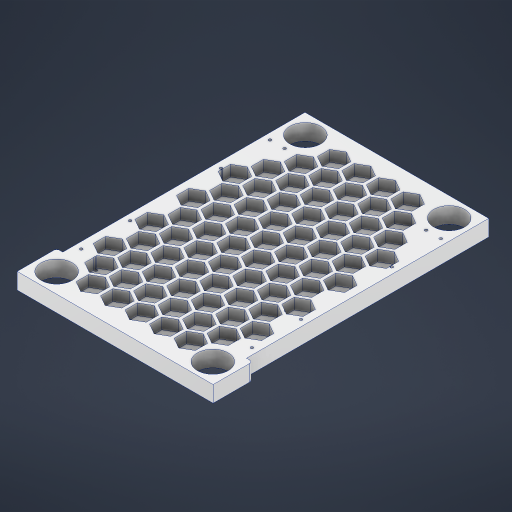
# Autodesk Inventor part: Weight Frame Top
Saved by Autodesk Inventor 2024 (Build 280153000, 153)
## iProperties
Created: 2022-10-18
Part Number: Weight Frame Top
Material: Aluminum 6061
Document SubType Name: Modeling
Designer: Hayden Swanson
Density: 2.7 g/cm^3
Appearance: Aluminum - Flat
Mass: 2392.19 g
Surface Area: 1313.96 cm^2
Volume: 885.998 cm^3
Author: Hayden Swanson
Autodesk Inventor part; units mm, degrees
ref_plane "YZ Plane" through (0, 0, 0) normal (1, 0, 0) x (0, 1, 0)
ref_plane "XZ Plane" through (0, 0, 0) normal (0, 1, 0) x (-1, 0, 0)
ref_plane "XY Plane" through (0, 0, 0) normal (0, 0, 1) x (1, 0, 0)
sketch "Sketch1" plane through (0, 0, 0) normal (0, 1, 0) x (-1, 0, 0)
  line L0 (0, 0) -> (190.5, 0)
  line L1 (190.5, 0) -> (190.5, -292.1)
  line L2 (190.5, -292.1) -> (0, -292.1)
  line L3 (0, -292.1) -> (0, 0)
  line L4 (0, -292.1) -> (-6.35, -292.1)
  line L5 (-6.35, -292.1) -> (-6.35, 0)
  line L6 (-6.35, 0) -> (0, 0)
  line L7 (190.5, -292.1) -> (196.85, -292.1)
  line L8 (196.85, -292.1) -> (196.85, 0)
  line L9 (196.85, 0) -> (190.5, 0)
  dimension "d0" = 190.5
  dimension "d1" = 292.1
  dimension "d259" = 6.35
  dimension "d260" = 6.35
  constraints: 20 end point, 4 perpendicular, 3 horizontal, 3 parallel
  measures "d0" distance of L1.end L2.end
  measures "d1" distance of L0.end L1.end
  measures "d259" distance of L2.end L4.end
  measures "d260" distance of L1.end L7.end
extrude "Extrusion1" add sketch "Sketch1" along normal blind 16.764
sketch "Sketch2" plane through (0, 16.764, 0) normal (0, 1, 0) x (1, 0, 0)
  line L0 (-176.2125, 0) -> (-176.2125, 20.32)
  line L1 (0, 0) -> (-14.2875, 0)
  line L2 (-14.2875, 0) -> (-14.2875, 20.32)
  line L3 (-190.5, 292.1) -> (-169.8625, 292.1)
  line L4 (-169.8625, 292.1) -> (-169.8625, 271.78)
  line L5 (-190.5, 271.78) -> (-190.5, 292.1)
  line L6 (0, 292.1) -> (-20.6375, 292.1)
  line L7 (-20.6375, 292.1) -> (-20.6375, 271.78)
  line L8 (0, 271.78) -> (0, 292.1)
  circle A0 centre (-176.2125, 20.32) radius 15.9766
  circle A1 centre (-14.2875, 20.32) radius 15.9766
  circle A2 centre (-20.6375, 271.78) radius 15.9766
  circle A3 centre (-169.8625, 271.78) radius 15.9766
  line L9 (6.35, 0) -> (6.35, 292.1) projected
  line L10 (6.35, 20.32) -> (-14.2875, 20.32)
  line L11 (-196.85, 292.1) -> (-196.85, 0) projected
  line L12 (-196.85, 20.32) -> (-176.2125, 20.32)
  dimension "d5" = 20.32
  dimension "d7" = 20.32
  dimension "d9" = 20.32
  dimension "d11" = 20.32
  dimension "d12" = 31.9532
  dimension "d14" = 31.9532
  dimension "d15" = 31.9532
  dimension "d264" = 31.9532
  dimension "d274" = 20.6375
  dimension "d276" = 20.6375
  constraints: 22 end point, 4 centre point, 4 coincident, 4 horizontal, 4 perpendicular, 2 parallel, 2 point on line
  measures "d5" distance of L0.end L0.start
  measures "d7" distance of L1.end L2.end
  measures "d9" distance of L3.end L4.end
  measures "d11" distance of L7.end L6.end
  measures "d12" diameter of A0
  measures "d14" diameter of A2
  measures "d15" diameter of A3
  measures "d264" diameter of A1
  measures "d274" distance of L10.start L10.end
  measures "d276" distance of L12.start L12.end
extrude "Extrusion2" cut sketch "Sketch2" against normal through all
sketch "Sketch7" plane through (0, 16.764, 0) normal (0, 1, 0) x (1, 0, 0)
  circle A0 centre (-14.2875, 20.32) radius 15.9766 projected
  line L0 (-14.2875, 53.2511) -> (-14.2875, 78.6511)
  line L1 (-14.2875, 78.6511) -> (-14.2875, 104.0511)
  line L2 (-14.2875, 53.2511) -> (-6.6675, 53.2511)
  line L3 (-14.2875, 104.0511) -> (-6.6675, 104.0511)
  line L4 (-14.2875, 104.0511) -> (-21.9075, 104.0511)
  line L5 (-14.2875, 53.2511) -> (-21.9075, 53.2511)
  line L6 (-14.2875, 198.2978) -> (-21.9075, 198.2978)
  line L7 (-14.2875, 249.0978) -> (-21.9075, 249.0978)
  line L8 (-14.2875, 198.2978) -> (-6.6675, 198.2978)
  line L9 (-14.2875, 249.0978) -> (-6.6675, 249.0978)
  circle A1 centre (-176.2125, 20.32) radius 15.9766 projected
  line L10 (-176.2125, 53.2511) -> (-176.2125, 78.6511)
  line L11 (-176.2125, 78.6511) -> (-176.2125, 104.0511)
  line L12 (-176.2125, 104.0511) -> (-176.2125, 198.2978)
  line L13 (-176.2125, 198.2978) -> (-176.2125, 223.6978)
  line L14 (-176.2125, 223.6978) -> (-176.2125, 249.0978)
  line L15 (-176.2125, 249.0978) -> (-168.5925, 249.0978)
  line L16 (-176.2125, 249.0978) -> (-183.8325, 249.0978)
  line L17 (-176.2125, 198.2978) -> (-183.8325, 198.2978)
  line L18 (-176.2125, 198.2978) -> (-168.5925, 198.2978)
  line L19 (-176.2125, 53.2511) -> (-183.8325, 53.2511)
  line L20 (-176.2125, 53.2511) -> (-168.5925, 53.2511)
  line L21 (-176.2125, 104.0511) -> (-183.8325, 104.0511)
  line L22 (-176.2125, 104.0511) -> (-168.5925, 104.0511)
  circle A2 centre (-183.8325, 53.2511) radius 1.75
  circle A3 centre (-183.8325, 104.0511) radius 1.75
  circle A4 centre (-168.5925, 53.2511) radius 1.75
  circle A5 centre (-168.5925, 104.0511) radius 1.75
  circle A6 centre (-183.8325, 198.2978) radius 1.75
  circle A7 centre (-168.5925, 198.2978) radius 1.75
  circle A8 centre (-183.8325, 249.0978) radius 1.75
  circle A9 centre (-168.5925, 249.0978) radius 1.75
  circle A10 centre (-21.9075, 53.2511) radius 1.75
  circle A11 centre (-6.6675, 53.2511) radius 1.75
  circle A12 centre (-21.9075, 104.0511) radius 1.75
  circle A13 centre (-6.6675, 104.0511) radius 1.75
  circle A14 centre (-21.9075, 198.2978) radius 1.75
  circle A15 centre (-21.9075, 249.0978) radius 1.75
  circle A16 centre (-6.6675, 198.2978) radius 1.75
  circle A17 centre (-6.6675, 249.0978) radius 1.75
  line L23 (-176.2125, 151.1745) -> (-14.2875, 151.1745)
  line L24 (-14.2875, 249.0978) -> (-14.2875, 53.2511)
  point P0 (0, 0)
  point P1 (6.35, 31.7989)
  point P2 (6.35, 8.8411)
  point P3 (-196.85, 8.8411)
  point P4 (-196.85, 31.7989)
  dimension "d167" = 25.4
  dimension "d168" = 25.4
  dimension "d169" = 94.2467
  dimension "d172" = 7.62
  dimension "d173" = 7.62
  dimension "d174" = 7.62
  dimension "d175" = 7.62
  dimension "d176" = 7.62
  dimension "d177" = 7.62
  dimension "d178" = 7.62
  dimension "d179" = 7.62
  dimension "d182" = 25.4
  dimension "d183" = 25.4
  dimension "d184" = 94.2467
  dimension "d185" = 25.4
  dimension "d186" = 25.4
  dimension "d187" = 7.62
  dimension "d188" = 7.62
  dimension "d189" = 7.62
  dimension "d190" = 7.62
  dimension "d191" = 7.62
  dimension "d192" = 7.62
  dimension "d193" = 7.62
  dimension "d194" = 7.62
  dimension "d195" = 3.5
  dimension "d196" = 3.5
  dimension "d197" = 3.5
  dimension "d198" = 3.5
  dimension "d199" = 3.5
  dimension "d200" = 3.5
  dimension "d201" = 3.5
  dimension "d202" = 3.5
  dimension "d203" = 3.5
  dimension "d204" = 3.5
  dimension "d205" = 3.5
  dimension "d206" = 3.5
  dimension "d207" = 3.5
  dimension "d208" = 3.5
  dimension "d209" = 3.5
  dimension "d210" = 3.5
  dimension "d258" = 161.925
  constraints: 50 end point, 16 centre point, 16 coincident, 14 horizontal, 4 point on line, 2 perpendicular, 1 midpoint, 2 other
  measures "d167" distance of L0.start L0.end
  measures "d168" distance of L0.end L1.end
  measures "d169" distance of L1.end L6.start
  measures "d172" distance of L0.start L2.end
  measures "d173" distance of L1.end L3.end
  measures "d174" distance of L1.end L4.end
  measures "d175" distance of L0.start L5.end
  measures "d176" distance of L6.start L6.end
  measures "d177" distance of L7.start L7.end
  measures "d178" distance of L6.start L8.end
  measures "d179" distance of L7.start L9.end
  measures "d182" distance of L10.start L10.end
  measures "d183" distance of L10.end L11.end
  measures "d184" distance of L11.end L12.end
  measures "d185" distance of L12.end L13.end
  measures "d186" distance of L13.end L14.end
  measures "d187" distance of L14.end L15.end
  measures "d188" distance of L14.end L16.end
  measures "d189" distance of L12.end L17.end
  measures "d190" distance of L12.end L18.end
  measures "d191" distance of L10.start L19.end
  measures "d192" distance of L10.start L20.end
  measures "d193" distance of L11.end L21.end
  measures "d194" distance of L11.end L22.end
  measures "d195" diameter of A2
  measures "d196" diameter of A3
  measures "d197" diameter of A4
  measures "d198" diameter of A5
  measures "d199" diameter of A6
  measures "d200" diameter of A7
  measures "d201" diameter of A8
  measures "d202" diameter of A9
  measures "d203" diameter of A10
  measures "d204" diameter of A11
  measures "d205" diameter of A12
  measures "d206" diameter of A13
  measures "d207" diameter of A14
  measures "d208" diameter of A15
  measures "d209" diameter of A16
  measures "d210" diameter of A17
  measures "d258" distance of L23.start L23.end
hole "Hole1" at (-183.8325, 16.764, -53.2511) at (-168.5925, 16.764, -53.2511) at (-183.8325, 16.764, -104.0511) at (-168.5925, 16.764, -104.0511) at (-183.8325, 16.764, -198.2978) at (-168.5925, 16.764, -198.2978) at (-183.8325, 16.764, -249.0978) at (-168.5925, 16.764, -249.0978) at (-6.6675, 16.764, -249.0978) at (-21.9075, 16.764, -249.0978) at (-6.6675, 16.764, -198.2978) at (-21.9075, 16.764, -198.2978) at (-6.6675, 16.764, -104.0511) at (-21.9075, 16.764, -104.0511) at (-6.6675, 16.764, -53.2511) at (-21.9075, 16.764, -53.2511) direction (0, -1, 0) diameter 2.85 end through all thread size "M3.5x0.6" class "6H" standard "ANSI Metric M Profile"
sketch "Sketch11" plane through (0, 16.764, 0) normal (0, 1, 0) x (1, 0, 0)
  circle A0 centre (-14.2875, 20.32) radius 15.9766 projected
  line L0 (-14.2875, 20.32) -> (-14.2875, 40.9575)
  line L1 (6.35, 292.1) -> (-196.85, 292.1) projected
  line L2 (6.35, 292.1) -> (0, 292.1)
  line L3 (0, 292.1) -> (0, 40.9575)
  line L4 (0, 40.9575) -> (6.35, 40.9575)
  line L5 (6.35, 40.9575) -> (6.35, 292.1)
  circle A1 centre (-176.2125, 20.32) radius 15.9766 projected
  line L6 (-176.2125, 20.32) -> (-176.2125, 40.9575)
  line L7 (-196.85, 292.1) -> (-196.85, 0) projected
  line L8 (-196.85, 292.1) -> (-190.5, 292.1)
  line L9 (-190.5, 292.1) -> (-190.5, 40.9575)
  line L10 (-190.5, 40.9575) -> (-196.85, 40.9575)
  line L11 (-196.85, 40.9575) -> (-196.85, 292.1)
  point P0 (0, 0)
  point P1 (-196.85, 40.9575)
  point P2 (6.35, 31.7989)
  point P3 (6.35, 8.8411)
  point P4 (-196.85, 8.8411)
  point P5 (-196.85, 31.7989)
  dimension "d266" = 20.6375
  dimension "d267" = 20.6375
  dimension "d272" = 6.35
  dimension "d273" = 6.35
  constraints: 20 end point, 4 parallel, 2 horizontal, 2 perpendicular, 2 vertical, 2 other
  measures "d266" distance of L0.start L0.end
  measures "d267" distance of L6.start L6.end
  measures "d272" distance of L3.end L4.end
  measures "d273" distance of L9.end L10.end
extrude "Extrusion10" cut sketch "Sketch11" against normal blind 16.764 contours L5 L4 L3 L1 | L9 L10 L7 L1
fillet "Fillet5" radius 3.175 2 edges at (-196.85, 8.382, -40.9575) (6.35, 8.382, -40.9575)
sketch "Sketch12" plane through (0, 16.764, 0) normal (0, 1, 0) x (1, 0, 0)
  line L0 (0, 292.1) -> (-190.5, 292.1) projected
  line L1 (0, 40.9575) -> (0, 292.1) projected
  arc A0 (-57.15, 292.1) -> (0, 234.95) centre (0, 292.1) ccw
  line L2 (-95.25, 316.441) -> (-95.25, -13.4796)
  line L3 (-232.3336, 146.05) -> (104.6921, 146.05)
  line L4 (-196.85, 0) -> (6.35, 0) projected
  arc A1 (-190.5, 234.95) -> (-133.35, 292.1) centre (-190.5, 292.1) ccw
  arc A2 (0, 57.15) -> (-57.15, 0) centre (0, 0) ccw
  arc A3 (-133.35, 0) -> (-190.5, 57.15) centre (-190.5, 0) ccw
  line L5 (-190.5, 234.95) -> (-190.5, 57.15)
  line L6 (-133.35, 0) -> (-57.15, 0)
  line L7 (0, 57.15) -> (0, 234.95)
  line L8 (-57.15, 292.1) -> (-133.35, 292.1)
  point P0 (0, 0)
  point P1 (-57.15, 0)
  dimension "d277" = 57.15
  dimension "d278" = 57.15
  dimension "d279" = 57.15
  dimension "d280" = 292.1
  dimension "d281" = 190.5
  dimension "d282" = 146.05
  dimension "d283" = 95.25
  constraints: 12 end point, 9 symmetric about line, 8 point on circle, 4 centre point, 3 collinear, 2 parallel, 2 point on line, 2 vertical, 1 horizontal, 3 other
  measures "d277" distance of L0.start L8.start
  measures "d278" distance of L0.start L7.end
  measures "d279" radius of A0
  measures "d280" distance between parallel lines of L0 L4
  measures "d281" distance of L0.end L0.start
  measures "d282" vertical distance of L0.end L3.start
  measures "d283" horizontal distance of L0.end L2.start
extrude "Extrusion11" [suppressed]
sketch "Sketch13" plane through (0, 16.764, 0) normal (0, 1, 0) x (1, 0, 0)
  line L0 (-160.4515, 34.036) -> (-160.4515, 21.336)
  line L1 (-160.4515, 21.336) -> (-171.45, 14.986)
  line L2 (-171.45, 14.986) -> (-182.4485, 21.336)
  line L3 (-182.4485, 21.336) -> (-182.4485, 34.036)
  line L4 (-182.4485, 34.036) -> (-171.45, 40.386)
  line L5 (-171.45, 40.386) -> (-160.4515, 34.036)
  line L6 (-190.5, 292.1) -> (-190.5, 40.9575) projected
  line L7 (-147.7515, 55.626) -> (-147.7515, 42.926)
  line L8 (-147.7515, 42.926) -> (-158.75, 36.576)
  line L9 (-158.75, 36.576) -> (-169.7485, 42.926)
  line L10 (-169.7485, 42.926) -> (-169.7485, 55.626)
  line L11 (-169.7485, 55.626) -> (-158.75, 61.976)
  line L12 (-158.75, 61.976) -> (-147.7515, 55.626)
  line L13 (-196.85, 0) -> (6.35, 0) projected
  line L14 (-147.7515, 86.106) -> (-158.75, 79.756)
  line L15 (-158.75, 79.756) -> (-169.7485, 86.106)
  line L16 (-147.7515, 98.806) -> (-147.7515, 86.106)
  line L17 (-169.7485, 86.106) -> (-169.7485, 98.806)
  line L18 (-169.7485, 98.806) -> (-158.75, 105.156)
  line L19 (-158.75, 105.156) -> (-147.7515, 98.806)
  line L20 (-182.4485, 77.216) -> (-171.45, 83.566)
  line L21 (-160.4515, 77.216) -> (-160.4515, 64.516)
  line L22 (-182.4485, 64.516) -> (-182.4485, 77.216)
  line L23 (-160.4515, 64.516) -> (-171.45, 58.166)
  line L24 (-171.45, 58.166) -> (-182.4485, 64.516)
  line L25 (-171.45, 83.566) -> (-160.4515, 77.216)
  line L26 (-147.7515, 129.286) -> (-158.75, 122.936)
  line L27 (-158.75, 122.936) -> (-169.7485, 129.286)
  line L28 (-147.7515, 141.986) -> (-147.7515, 129.286)
  line L29 (-169.7485, 129.286) -> (-169.7485, 141.986)
  line L30 (-169.7485, 141.986) -> (-158.75, 148.336)
  line L31 (-158.75, 148.336) -> (-147.7515, 141.986)
  line L32 (-182.4485, 120.396) -> (-171.45, 126.746)
  line L33 (-160.4515, 120.396) -> (-160.4515, 107.696)
  line L34 (-182.4485, 107.696) -> (-182.4485, 120.396)
  line L35 (-160.4515, 107.696) -> (-171.45, 101.346)
  line L36 (-171.45, 101.346) -> (-182.4485, 107.696)
  line L37 (-171.45, 126.746) -> (-160.4515, 120.396)
  line L38 (-147.7515, 172.466) -> (-158.75, 166.116)
  line L39 (-158.75, 166.116) -> (-169.7485, 172.466)
  line L40 (-147.7515, 185.166) -> (-147.7515, 172.466)
  line L41 (-169.7485, 172.466) -> (-169.7485, 185.166)
  line L42 (-169.7485, 185.166) -> (-158.75, 191.516)
  line L43 (-158.75, 191.516) -> (-147.7515, 185.166)
  line L44 (-182.4485, 163.576) -> (-171.45, 169.926)
  line L45 (-160.4515, 163.576) -> (-160.4515, 150.876)
  line L46 (-182.4485, 150.876) -> (-182.4485, 163.576)
  line L47 (-160.4515, 150.876) -> (-171.45, 144.526)
  line L48 (-171.45, 144.526) -> (-182.4485, 150.876)
  line L49 (-171.45, 169.926) -> (-160.4515, 163.576)
  line L50 (-147.7515, 215.646) -> (-158.75, 209.296)
  line L51 (-158.75, 209.296) -> (-169.7485, 215.646)
  line L52 (-147.7515, 228.346) -> (-147.7515, 215.646)
  line L53 (-169.7485, 215.646) -> (-169.7485, 228.346)
  line L54 (-169.7485, 228.346) -> (-158.75, 234.696)
  line L55 (-158.75, 234.696) -> (-147.7515, 228.346)
  line L56 (-182.4485, 206.756) -> (-171.45, 213.106)
  line L57 (-160.4515, 206.756) -> (-160.4515, 194.056)
  line L58 (-182.4485, 194.056) -> (-182.4485, 206.756)
  line L59 (-160.4515, 194.056) -> (-171.45, 187.706)
  line L60 (-171.45, 187.706) -> (-182.4485, 194.056)
  line L61 (-171.45, 213.106) -> (-160.4515, 206.756)
  line L62 (-122.3515, 42.926) -> (-133.35, 36.576)
  line L63 (-133.35, 36.576) -> (-144.3485, 42.926)
  line L64 (-122.3515, 55.626) -> (-122.3515, 42.926)
  line L65 (-144.3485, 42.926) -> (-144.3485, 55.626)
  line L66 (-144.3485, 55.626) -> (-133.35, 61.976)
  line L67 (-133.35, 61.976) -> (-122.3515, 55.626)
  line L68 (-157.0485, 34.036) -> (-146.05, 40.386)
  line L69 (-135.0515, 34.036) -> (-135.0515, 21.336)
  line L70 (-157.0485, 21.336) -> (-157.0485, 34.036)
  line L71 (-135.0515, 21.336) -> (-146.05, 14.986)
  line L72 (-146.05, 14.986) -> (-157.0485, 21.336)
  line L73 (-146.05, 40.386) -> (-135.0515, 34.036)
  line L74 (-122.3515, 86.106) -> (-133.35, 79.756)
  line L75 (-133.35, 79.756) -> (-144.3485, 86.106)
  line L76 (-122.3515, 98.806) -> (-122.3515, 86.106)
  line L77 (-144.3485, 86.106) -> (-144.3485, 98.806)
  line L78 (-144.3485, 98.806) -> (-133.35, 105.156)
  line L79 (-133.35, 105.156) -> (-122.3515, 98.806)
  line L80 (-157.0485, 77.216) -> (-146.05, 83.566)
  line L81 (-135.0515, 77.216) -> (-135.0515, 64.516)
  line L82 (-157.0485, 64.516) -> (-157.0485, 77.216)
  line L83 (-135.0515, 64.516) -> (-146.05, 58.166)
  line L84 (-146.05, 58.166) -> (-157.0485, 64.516)
  line L85 (-146.05, 83.566) -> (-135.0515, 77.216)
  line L86 (-122.3515, 129.286) -> (-133.35, 122.936)
  line L87 (-133.35, 122.936) -> (-144.3485, 129.286)
  line L88 (-122.3515, 141.986) -> (-122.3515, 129.286)
  line L89 (-144.3485, 129.286) -> (-144.3485, 141.986)
  line L90 (-144.3485, 141.986) -> (-133.35, 148.336)
  line L91 (-133.35, 148.336) -> (-122.3515, 141.986)
  line L92 (-157.0485, 120.396) -> (-146.05, 126.746)
  line L93 (-135.0515, 120.396) -> (-135.0515, 107.696)
  line L94 (-157.0485, 107.696) -> (-157.0485, 120.396)
  line L95 (-135.0515, 107.696) -> (-146.05, 101.346)
  line L96 (-146.05, 101.346) -> (-157.0485, 107.696)
  line L97 (-146.05, 126.746) -> (-135.0515, 120.396)
  line L98 (-122.3515, 172.466) -> (-133.35, 166.116)
  line L99 (-133.35, 166.116) -> (-144.3485, 172.466)
  line L100 (-122.3515, 185.166) -> (-122.3515, 172.466)
  line L101 (-144.3485, 172.466) -> (-144.3485, 185.166)
  line L102 (-144.3485, 185.166) -> (-133.35, 191.516)
  line L103 (-133.35, 191.516) -> (-122.3515, 185.166)
  line L104 (-157.0485, 163.576) -> (-146.05, 169.926)
  line L105 (-135.0515, 163.576) -> (-135.0515, 150.876)
  line L106 (-157.0485, 150.876) -> (-157.0485, 163.576)
  line L107 (-135.0515, 150.876) -> (-146.05, 144.526)
  line L108 (-146.05, 144.526) -> (-157.0485, 150.876)
  line L109 (-146.05, 169.926) -> (-135.0515, 163.576)
  line L110 (-122.3515, 215.646) -> (-133.35, 209.296)
  line L111 (-133.35, 209.296) -> (-144.3485, 215.646)
  line L112 (-122.3515, 228.346) -> (-122.3515, 215.646)
  line L113 (-144.3485, 215.646) -> (-144.3485, 228.346)
  line L114 (-144.3485, 228.346) -> (-133.35, 234.696)
  line L115 (-133.35, 234.696) -> (-122.3515, 228.346)
  line L116 (-157.0485, 206.756) -> (-146.05, 213.106)
  line L117 (-135.0515, 206.756) -> (-135.0515, 194.056)
  line L118 (-157.0485, 194.056) -> (-157.0485, 206.756)
  line L119 (-135.0515, 194.056) -> (-146.05, 187.706)
  line L120 (-146.05, 187.706) -> (-157.0485, 194.056)
  line L121 (-146.05, 213.106) -> (-135.0515, 206.756)
  line L122 (-96.9515, 42.926) -> (-107.95, 36.576)
  line L123 (-107.95, 36.576) -> (-118.9485, 42.926)
  line L124 (-96.9515, 55.626) -> (-96.9515, 42.926)
  line L125 (-118.9485, 42.926) -> (-118.9485, 55.626)
  line L126 (-118.9485, 55.626) -> (-107.95, 61.976)
  line L127 (-107.95, 61.976) -> (-96.9515, 55.626)
  line L128 (-131.6485, 34.036) -> (-120.65, 40.386)
  line L129 (-109.6515, 34.036) -> (-109.6515, 21.336)
  line L130 (-131.6485, 21.336) -> (-131.6485, 34.036)
  line L131 (-109.6515, 21.336) -> (-120.65, 14.986)
  line L132 (-120.65, 14.986) -> (-131.6485, 21.336)
  line L133 (-120.65, 40.386) -> (-109.6515, 34.036)
  line L134 (-96.9515, 86.106) -> (-107.95, 79.756)
  line L135 (-107.95, 79.756) -> (-118.9485, 86.106)
  line L136 (-96.9515, 98.806) -> (-96.9515, 86.106)
  line L137 (-118.9485, 86.106) -> (-118.9485, 98.806)
  line L138 (-118.9485, 98.806) -> (-107.95, 105.156)
  line L139 (-107.95, 105.156) -> (-96.9515, 98.806)
  line L140 (-131.6485, 77.216) -> (-120.65, 83.566)
  line L141 (-109.6515, 77.216) -> (-109.6515, 64.516)
  line L142 (-131.6485, 64.516) -> (-131.6485, 77.216)
  line L143 (-109.6515, 64.516) -> (-120.65, 58.166)
  line L144 (-120.65, 58.166) -> (-131.6485, 64.516)
  line L145 (-120.65, 83.566) -> (-109.6515, 77.216)
  line L146 (-96.9515, 129.286) -> (-107.95, 122.936)
  line L147 (-107.95, 122.936) -> (-118.9485, 129.286)
  line L148 (-96.9515, 141.986) -> (-96.9515, 129.286)
  line L149 (-118.9485, 129.286) -> (-118.9485, 141.986)
  line L150 (-118.9485, 141.986) -> (-107.95, 148.336)
  line L151 (-107.95, 148.336) -> (-96.9515, 141.986)
  line L152 (-131.6485, 120.396) -> (-120.65, 126.746)
  line L153 (-109.6515, 120.396) -> (-109.6515, 107.696)
  line L154 (-131.6485, 107.696) -> (-131.6485, 120.396)
  line L155 (-109.6515, 107.696) -> (-120.65, 101.346)
  line L156 (-120.65, 101.346) -> (-131.6485, 107.696)
  line L157 (-120.65, 126.746) -> (-109.6515, 120.396)
  line L158 (-96.9515, 172.466) -> (-107.95, 166.116)
  line L159 (-107.95, 166.116) -> (-118.9485, 172.466)
  line L160 (-96.9515, 185.166) -> (-96.9515, 172.466)
  line L161 (-118.9485, 172.466) -> (-118.9485, 185.166)
  line L162 (-118.9485, 185.166) -> (-107.95, 191.516)
  line L163 (-107.95, 191.516) -> (-96.9515, 185.166)
  line L164 (-131.6485, 163.576) -> (-120.65, 169.926)
  line L165 (-109.6515, 163.576) -> (-109.6515, 150.876)
  line L166 (-131.6485, 150.876) -> (-131.6485, 163.576)
  line L167 (-109.6515, 150.876) -> (-120.65, 144.526)
  line L168 (-120.65, 144.526) -> (-131.6485, 150.876)
  line L169 (-120.65, 169.926) -> (-109.6515, 163.576)
  line L170 (-96.9515, 215.646) -> (-107.95, 209.296)
  line L171 (-107.95, 209.296) -> (-118.9485, 215.646)
  line L172 (-96.9515, 228.346) -> (-96.9515, 215.646)
  line L173 (-118.9485, 215.646) -> (-118.9485, 228.346)
  line L174 (-118.9485, 228.346) -> (-107.95, 234.696)
  line L175 (-107.95, 234.696) -> (-96.9515, 228.346)
  line L176 (-131.6485, 206.756) -> (-120.65, 213.106)
  line L177 (-109.6515, 206.756) -> (-109.6515, 194.056)
  line L178 (-131.6485, 194.056) -> (-131.6485, 206.756)
  line L179 (-109.6515, 194.056) -> (-120.65, 187.706)
  line L180 (-120.65, 187.706) -> (-131.6485, 194.056)
  line L181 (-120.65, 213.106) -> (-109.6515, 206.756)
  line L182 (-71.5515, 42.926) -> (-82.55, 36.576)
  line L183 (-82.55, 36.576) -> (-93.5485, 42.926)
  line L184 (-71.5515, 55.626) -> (-71.5515, 42.926)
  line L185 (-93.5485, 42.926) -> (-93.5485, 55.626)
  line L186 (-93.5485, 55.626) -> (-82.55, 61.976)
  line L187 (-82.55, 61.976) -> (-71.5515, 55.626)
  line L188 (-106.2485, 34.036) -> (-95.25, 40.386)
  line L189 (-84.2515, 34.036) -> (-84.2515, 21.336)
  line L190 (-106.2485, 21.336) -> (-106.2485, 34.036)
  line L191 (-84.2515, 21.336) -> (-95.25, 14.986)
  line L192 (-95.25, 14.986) -> (-106.2485, 21.336)
  line L193 (-95.25, 40.386) -> (-84.2515, 34.036)
  line L194 (-71.5515, 86.106) -> (-82.55, 79.756)
  line L195 (-82.55, 79.756) -> (-93.5485, 86.106)
  line L196 (-71.5515, 98.806) -> (-71.5515, 86.106)
  line L197 (-93.5485, 86.106) -> (-93.5485, 98.806)
  line L198 (-93.5485, 98.806) -> (-82.55, 105.156)
  line L199 (-82.55, 105.156) -> (-71.5515, 98.806)
  line L200 (-106.2485, 77.216) -> (-95.25, 83.566)
  line L201 (-84.2515, 77.216) -> (-84.2515, 64.516)
  line L202 (-106.2485, 64.516) -> (-106.2485, 77.216)
  line L203 (-84.2515, 64.516) -> (-95.25, 58.166)
  line L204 (-95.25, 58.166) -> (-106.2485, 64.516)
  line L205 (-95.25, 83.566) -> (-84.2515, 77.216)
  line L206 (-71.5515, 129.286) -> (-82.55, 122.936)
  line L207 (-82.55, 122.936) -> (-93.5485, 129.286)
  line L208 (-71.5515, 141.986) -> (-71.5515, 129.286)
  line L209 (-93.5485, 129.286) -> (-93.5485, 141.986)
  line L210 (-93.5485, 141.986) -> (-82.55, 148.336)
  line L211 (-82.55, 148.336) -> (-71.5515, 141.986)
  line L212 (-106.2485, 120.396) -> (-95.25, 126.746)
  line L213 (-84.2515, 120.396) -> (-84.2515, 107.696)
  line L214 (-106.2485, 107.696) -> (-106.2485, 120.396)
  line L215 (-84.2515, 107.696) -> (-95.25, 101.346)
  line L216 (-95.25, 101.346) -> (-106.2485, 107.696)
  line L217 (-95.25, 126.746) -> (-84.2515, 120.396)
  line L218 (-71.5515, 172.466) -> (-82.55, 166.116)
  line L219 (-82.55, 166.116) -> (-93.5485, 172.466)
  line L220 (-71.5515, 185.166) -> (-71.5515, 172.466)
  line L221 (-93.5485, 172.466) -> (-93.5485, 185.166)
  line L222 (-93.5485, 185.166) -> (-82.55, 191.516)
  line L223 (-82.55, 191.516) -> (-71.5515, 185.166)
  line L224 (-106.2485, 163.576) -> (-95.25, 169.926)
  line L225 (-84.2515, 163.576) -> (-84.2515, 150.876)
  line L226 (-106.2485, 150.876) -> (-106.2485, 163.576)
  line L227 (-84.2515, 150.876) -> (-95.25, 144.526)
  line L228 (-95.25, 144.526) -> (-106.2485, 150.876)
  line L229 (-95.25, 169.926) -> (-84.2515, 163.576)
  line L230 (-71.5515, 215.646) -> (-82.55, 209.296)
  line L231 (-82.55, 209.296) -> (-93.5485, 215.646)
  line L232 (-71.5515, 228.346) -> (-71.5515, 215.646)
  line L233 (-93.5485, 215.646) -> (-93.5485, 228.346)
  line L234 (-93.5485, 228.346) -> (-82.55, 234.696)
  line L235 (-82.55, 234.696) -> (-71.5515, 228.346)
  line L236 (-106.2485, 206.756) -> (-95.25, 213.106)
  line L237 (-84.2515, 206.756) -> (-84.2515, 194.056)
  line L238 (-106.2485, 194.056) -> (-106.2485, 206.756)
  line L239 (-84.2515, 194.056) -> (-95.25, 187.706)
  line L240 (-95.25, 187.706) -> (-106.2485, 194.056)
  line L241 (-95.25, 213.106) -> (-84.2515, 206.756)
  line L242 (-46.1515, 42.926) -> (-57.15, 36.576)
  line L243 (-57.15, 36.576) -> (-68.1485, 42.926)
  line L244 (-46.1515, 55.626) -> (-46.1515, 42.926)
  line L245 (-68.1485, 42.926) -> (-68.1485, 55.626)
  line L246 (-68.1485, 55.626) -> (-57.15, 61.976)
  line L247 (-57.15, 61.976) -> (-46.1515, 55.626)
  line L248 (-80.8485, 34.036) -> (-69.85, 40.386)
  line L249 (-58.8515, 34.036) -> (-58.8515, 21.336)
  line L250 (-80.8485, 21.336) -> (-80.8485, 34.036)
  line L251 (-58.8515, 21.336) -> (-69.85, 14.986)
  line L252 (-69.85, 14.986) -> (-80.8485, 21.336)
  line L253 (-69.85, 40.386) -> (-58.8515, 34.036)
  line L254 (-46.1515, 86.106) -> (-57.15, 79.756)
  line L255 (-57.15, 79.756) -> (-68.1485, 86.106)
  line L256 (-46.1515, 98.806) -> (-46.1515, 86.106)
  line L257 (-68.1485, 86.106) -> (-68.1485, 98.806)
  line L258 (-68.1485, 98.806) -> (-57.15, 105.156)
  line L259 (-57.15, 105.156) -> (-46.1515, 98.806)
  line L260 (-80.8485, 77.216) -> (-69.85, 83.566)
  line L261 (-58.8515, 77.216) -> (-58.8515, 64.516)
  line L262 (-80.8485, 64.516) -> (-80.8485, 77.216)
  line L263 (-58.8515, 64.516) -> (-69.85, 58.166)
  line L264 (-69.85, 58.166) -> (-80.8485, 64.516)
  line L265 (-69.85, 83.566) -> (-58.8515, 77.216)
  line L266 (-46.1515, 129.286) -> (-57.15, 122.936)
  line L267 (-57.15, 122.936) -> (-68.1485, 129.286)
  line L268 (-46.1515, 141.986) -> (-46.1515, 129.286)
  line L269 (-68.1485, 129.286) -> (-68.1485, 141.986)
  line L270 (-68.1485, 141.986) -> (-57.15, 148.336)
  line L271 (-57.15, 148.336) -> (-46.1515, 141.986)
  line L272 (-80.8485, 120.396) -> (-69.85, 126.746)
  line L273 (-58.8515, 120.396) -> (-58.8515, 107.696)
  line L274 (-80.8485, 107.696) -> (-80.8485, 120.396)
  line L275 (-58.8515, 107.696) -> (-69.85, 101.346)
  line L276 (-69.85, 101.346) -> (-80.8485, 107.696)
  line L277 (-69.85, 126.746) -> (-58.8515, 120.396)
  line L278 (-46.1515, 172.466) -> (-57.15, 166.116)
  line L279 (-57.15, 166.116) -> (-68.1485, 172.466)
  line L280 (-46.1515, 185.166) -> (-46.1515, 172.466)
  line L281 (-68.1485, 172.466) -> (-68.1485, 185.166)
  line L282 (-68.1485, 185.166) -> (-57.15, 191.516)
  line L283 (-57.15, 191.516) -> (-46.1515, 185.166)
  line L284 (-80.8485, 163.576) -> (-69.85, 169.926)
  line L285 (-58.8515, 163.576) -> (-58.8515, 150.876)
  line L286 (-80.8485, 150.876) -> (-80.8485, 163.576)
  line L287 (-58.8515, 150.876) -> (-69.85, 144.526)
  line L288 (-69.85, 144.526) -> (-80.8485, 150.876)
  line L289 (-69.85, 169.926) -> (-58.8515, 163.576)
  line L290 (-46.1515, 215.646) -> (-57.15, 209.296)
  line L291 (-57.15, 209.296) -> (-68.1485, 215.646)
  line L292 (-46.1515, 228.346) -> (-46.1515, 215.646)
  line L293 (-68.1485, 215.646) -> (-68.1485, 228.346)
  line L294 (-68.1485, 228.346) -> (-57.15, 234.696)
  line L295 (-57.15, 234.696) -> (-46.1515, 228.346)
  line L296 (-80.8485, 206.756) -> (-69.85, 213.106)
  line L297 (-58.8515, 206.756) -> (-58.8515, 194.056)
  line L298 (-80.8485, 194.056) -> (-80.8485, 206.756)
  line L299 (-58.8515, 194.056) -> (-69.85, 187.706)
  line L300 (-69.85, 187.706) -> (-80.8485, 194.056)
  line L301 (-69.85, 213.106) -> (-58.8515, 206.756)
  line L302 (-20.7515, 42.926) -> (-31.75, 36.576)
  line L303 (-31.75, 36.576) -> (-42.7485, 42.926)
  line L304 (-20.7515, 55.626) -> (-20.7515, 42.926)
  line L305 (-42.7485, 42.926) -> (-42.7485, 55.626)
  line L306 (-42.7485, 55.626) -> (-31.75, 61.976)
  line L307 (-31.75, 61.976) -> (-20.7515, 55.626)
  line L308 (-55.4485, 34.036) -> (-44.45, 40.386)
  line L309 (-33.4515, 34.036) -> (-33.4515, 21.336)
  line L310 (-55.4485, 21.336) -> (-55.4485, 34.036)
  line L311 (-33.4515, 21.336) -> (-44.45, 14.986)
  line L312 (-44.45, 14.986) -> (-55.4485, 21.336)
  line L313 (-44.45, 40.386) -> (-33.4515, 34.036)
  line L314 (-20.7515, 86.106) -> (-31.75, 79.756)
  line L315 (-31.75, 79.756) -> (-42.7485, 86.106)
  line L316 (-20.7515, 98.806) -> (-20.7515, 86.106)
  line L317 (-42.7485, 86.106) -> (-42.7485, 98.806)
  line L318 (-42.7485, 98.806) -> (-31.75, 105.156)
  line L319 (-31.75, 105.156) -> (-20.7515, 98.806)
  line L320 (-55.4485, 77.216) -> (-44.45, 83.566)
  line L321 (-33.4515, 77.216) -> (-33.4515, 64.516)
  line L322 (-55.4485, 64.516) -> (-55.4485, 77.216)
  line L323 (-33.4515, 64.516) -> (-44.45, 58.166)
  line L324 (-44.45, 58.166) -> (-55.4485, 64.516)
  line L325 (-44.45, 83.566) -> (-33.4515, 77.216)
  line L326 (-20.7515, 129.286) -> (-31.75, 122.936)
  line L327 (-31.75, 122.936) -> (-42.7485, 129.286)
  line L328 (-20.7515, 141.986) -> (-20.7515, 129.286)
  line L329 (-42.7485, 129.286) -> (-42.7485, 141.986)
  line L330 (-42.7485, 141.986) -> (-31.75, 148.336)
  line L331 (-31.75, 148.336) -> (-20.7515, 141.986)
  line L332 (-55.4485, 120.396) -> (-44.45, 126.746)
  line L333 (-33.4515, 120.396) -> (-33.4515, 107.696)
  line L334 (-55.4485, 107.696) -> (-55.4485, 120.396)
  line L335 (-33.4515, 107.696) -> (-44.45, 101.346)
  line L336 (-44.45, 101.346) -> (-55.4485, 107.696)
  line L337 (-44.45, 126.746) -> (-33.4515, 120.396)
  line L338 (-20.7515, 172.466) -> (-31.75, 166.116)
  line L339 (-31.75, 166.116) -> (-42.7485, 172.466)
  line L340 (-20.7515, 185.166) -> (-20.7515, 172.466)
  line L341 (-42.7485, 172.466) -> (-42.7485, 185.166)
  line L342 (-42.7485, 185.166) -> (-31.75, 191.516)
  line L343 (-31.75, 191.516) -> (-20.7515, 185.166)
  line L344 (-55.4485, 163.576) -> (-44.45, 169.926)
  line L345 (-33.4515, 163.576) -> (-33.4515, 150.876)
  line L346 (-55.4485, 150.876) -> (-55.4485, 163.576)
  line L347 (-33.4515, 150.876) -> (-44.45, 144.526)
  line L348 (-44.45, 144.526) -> (-55.4485, 150.876)
  line L349 (-44.45, 169.926) -> (-33.4515, 163.576)
  line L350 (-20.7515, 215.646) -> (-31.75, 209.296)
  line L351 (-31.75, 209.296) -> (-42.7485, 215.646)
  line L352 (-20.7515, 228.346) -> (-20.7515, 215.646)
  line L353 (-42.7485, 215.646) -> (-42.7485, 228.346)
  line L354 (-42.7485, 228.346) -> (-31.75, 234.696)
  line L355 (-31.75, 234.696) -> (-20.7515, 228.346)
  line L356 (-55.4485, 206.756) -> (-44.45, 213.106)
  line L357 (-33.4515, 206.756) -> (-33.4515, 194.056)
  line L358 (-55.4485, 194.056) -> (-55.4485, 206.756)
  line L359 (-33.4515, 194.056) -> (-44.45, 187.706)
  line L360 (-44.45, 187.706) -> (-55.4485, 194.056)
  line L361 (-44.45, 213.106) -> (-33.4515, 206.756)
  line L362 (-147.7515, 258.826) -> (-158.75, 252.476)
  line L363 (-158.75, 252.476) -> (-169.7485, 258.826)
  line L364 (-147.7515, 271.526) -> (-147.7515, 258.826)
  line L365 (-169.7485, 258.826) -> (-169.7485, 271.526)
  line L366 (-169.7485, 271.526) -> (-158.75, 277.876)
  line L367 (-158.75, 277.876) -> (-147.7515, 271.526)
  line L368 (-182.4485, 249.936) -> (-171.45, 256.286)
  line L369 (-160.4515, 249.936) -> (-160.4515, 237.236)
  line L370 (-182.4485, 237.236) -> (-182.4485, 249.936)
  line L371 (-160.4515, 237.236) -> (-171.45, 230.886)
  line L372 (-171.45, 230.886) -> (-182.4485, 237.236)
  line L373 (-171.45, 256.286) -> (-160.4515, 249.936)
  line L374 (-122.3515, 258.826) -> (-133.35, 252.476)
  line L375 (-133.35, 252.476) -> (-144.3485, 258.826)
  line L376 (-122.3515, 271.526) -> (-122.3515, 258.826)
  line L377 (-144.3485, 258.826) -> (-144.3485, 271.526)
  line L378 (-144.3485, 271.526) -> (-133.35, 277.876)
  line L379 (-133.35, 277.876) -> (-122.3515, 271.526)
  line L380 (-157.0485, 249.936) -> (-146.05, 256.286)
  line L381 (-135.0515, 249.936) -> (-135.0515, 237.236)
  line L382 (-157.0485, 237.236) -> (-157.0485, 249.936)
  line L383 (-135.0515, 237.236) -> (-146.05, 230.886)
  line L384 (-146.05, 230.886) -> (-157.0485, 237.236)
  line L385 (-146.05, 256.286) -> (-135.0515, 249.936)
  line L386 (-96.9515, 258.826) -> (-107.95, 252.476)
  line L387 (-107.95, 252.476) -> (-118.9485, 258.826)
  line L388 (-96.9515, 271.526) -> (-96.9515, 258.826)
  line L389 (-118.9485, 258.826) -> (-118.9485, 271.526)
  line L390 (-118.9485, 271.526) -> (-107.95, 277.876)
  line L391 (-107.95, 277.876) -> (-96.9515, 271.526)
  line L392 (-131.6485, 249.936) -> (-120.65, 256.286)
  line L393 (-109.6515, 249.936) -> (-109.6515, 237.236)
  line L394 (-131.6485, 237.236) -> (-131.6485, 249.936)
  line L395 (-109.6515, 237.236) -> (-120.65, 230.886)
  line L396 (-120.65, 230.886) -> (-131.6485, 237.236)
  line L397 (-120.65, 256.286) -> (-109.6515, 249.936)
  line L398 (-71.5515, 258.826) -> (-82.55, 252.476)
  line L399 (-82.55, 252.476) -> (-93.5485, 258.826)
  line L400 (-71.5515, 271.526) -> (-71.5515, 258.826)
  line L401 (-93.5485, 258.826) -> (-93.5485, 271.526)
  line L402 (-93.5485, 271.526) -> (-82.55, 277.876)
  line L403 (-82.55, 277.876) -> (-71.5515, 271.526)
  line L404 (-106.2485, 249.936) -> (-95.25, 256.286)
  line L405 (-84.2515, 249.936) -> (-84.2515, 237.236)
  line L406 (-106.2485, 237.236) -> (-106.2485, 249.936)
  line L407 (-84.2515, 237.236) -> (-95.25, 230.886)
  line L408 (-95.25, 230.886) -> (-106.2485, 237.236)
  line L409 (-95.25, 256.286) -> (-84.2515, 249.936)
  line L410 (-46.1515, 258.826) -> (-57.15, 252.476)
  line L411 (-57.15, 252.476) -> (-68.1485, 258.826)
  line L412 (-46.1515, 271.526) -> (-46.1515, 258.826)
  line L413 (-68.1485, 258.826) -> (-68.1485, 271.526)
  line L414 (-68.1485, 271.526) -> (-57.15, 277.876)
  line L415 (-57.15, 277.876) -> (-46.1515, 271.526)
  line L416 (-80.8485, 249.936) -> (-69.85, 256.286)
  line L417 (-58.8515, 249.936) -> (-58.8515, 237.236)
  line L418 (-80.8485, 237.236) -> (-80.8485, 249.936)
  line L419 (-58.8515, 237.236) -> (-69.85, 230.886)
  line L420 (-69.85, 230.886) -> (-80.8485, 237.236)
  line L421 (-69.85, 256.286) -> (-58.8515, 249.936)
  line L422 (-20.7515, 258.826) -> (-31.75, 252.476)
  line L423 (-31.75, 252.476) -> (-42.7485, 258.826)
  line L424 (-20.7515, 271.526) -> (-20.7515, 258.826)
  line L425 (-42.7485, 258.826) -> (-42.7485, 271.526)
  line L426 (-42.7485, 271.526) -> (-31.75, 277.876)
  line L427 (-31.75, 277.876) -> (-20.7515, 271.526)
  line L428 (-55.4485, 249.936) -> (-44.45, 256.286)
  line L429 (-33.4515, 249.936) -> (-33.4515, 237.236)
  line L430 (-55.4485, 237.236) -> (-55.4485, 249.936)
  line L431 (-33.4515, 237.236) -> (-44.45, 230.886)
  line L432 (-44.45, 230.886) -> (-55.4485, 237.236)
  line L433 (-44.45, 256.286) -> (-33.4515, 249.936)
  circle A0 centre (-14.2875, 20.32) radius 15.9766 projected
  circle A1 centre (-176.2125, 20.32) radius 15.9766 projected
  line L434 (4.6485, 42.926) -> (-6.35, 36.576)
  line L435 (-6.35, 36.576) -> (-17.3485, 42.926)
  line L436 (4.6485, 55.626) -> (4.6485, 42.926)
  line L437 (-17.3485, 42.926) -> (-17.3485, 55.626)
  line L438 (-17.3485, 55.626) -> (-6.35, 61.976)
  line L439 (-6.35, 61.976) -> (4.6485, 55.626)
  line L440 (-30.0485, 34.036) -> (-19.05, 40.386)
  line L441 (-8.0515, 34.036) -> (-8.0515, 21.336)
  line L442 (-30.0485, 21.336) -> (-30.0485, 34.036)
  line L443 (-8.0515, 21.336) -> (-19.05, 14.986)
  line L444 (-19.05, 14.986) -> (-30.0485, 21.336)
  line L445 (-19.05, 40.386) -> (-8.0515, 34.036)
  line L446 (4.6485, 86.106) -> (-6.35, 79.756)
  line L447 (-6.35, 79.756) -> (-17.3485, 86.106)
  line L448 (4.6485, 98.806) -> (4.6485, 86.106)
  line L449 (-17.3485, 86.106) -> (-17.3485, 98.806)
  line L450 (-17.3485, 98.806) -> (-6.35, 105.156)
  line L451 (-6.35, 105.156) -> (4.6485, 98.806)
  line L452 (-30.0485, 77.216) -> (-19.05, 83.566)
  line L453 (-8.0515, 77.216) -> (-8.0515, 64.516)
  line L454 (-30.0485, 64.516) -> (-30.0485, 77.216)
  line L455 (-8.0515, 64.516) -> (-19.05, 58.166)
  line L456 (-19.05, 58.166) -> (-30.0485, 64.516)
  line L457 (-19.05, 83.566) -> (-8.0515, 77.216)
  line L458 (4.6485, 129.286) -> (-6.35, 122.936)
  line L459 (-6.35, 122.936) -> (-17.3485, 129.286)
  line L460 (4.6485, 141.986) -> (4.6485, 129.286)
  line L461 (-17.3485, 129.286) -> (-17.3485, 141.986)
  line L462 (-17.3485, 141.986) -> (-6.35, 148.336)
  line L463 (-6.35, 148.336) -> (4.6485, 141.986)
  line L464 (-30.0485, 120.396) -> (-19.05, 126.746)
  line L465 (-8.0515, 120.396) -> (-8.0515, 107.696)
  line L466 (-30.0485, 107.696) -> (-30.0485, 120.396)
  line L467 (-8.0515, 107.696) -> (-19.05, 101.346)
  line L468 (-19.05, 101.346) -> (-30.0485, 107.696)
  line L469 (-19.05, 126.746) -> (-8.0515, 120.396)
  line L470 (4.6485, 172.466) -> (-6.35, 166.116)
  line L471 (-6.35, 166.116) -> (-17.3485, 172.466)
  line L472 (4.6485, 185.166) -> (4.6485, 172.466)
  line L473 (-17.3485, 172.466) -> (-17.3485, 185.166)
  line L474 (-17.3485, 185.166) -> (-6.35, 191.516)
  line L475 (-6.35, 191.516) -> (4.6485, 185.166)
  line L476 (-30.0485, 163.576) -> (-19.05, 169.926)
  line L477 (-8.0515, 163.576) -> (-8.0515, 150.876)
  line L478 (-30.0485, 150.876) -> (-30.0485, 163.576)
  line L479 (-8.0515, 150.876) -> (-19.05, 144.526)
  line L480 (-19.05, 144.526) -> (-30.0485, 150.876)
  line L481 (-19.05, 169.926) -> (-8.0515, 163.576)
  line L482 (4.6485, 215.646) -> (-6.35, 209.296)
  line L483 (-6.35, 209.296) -> (-17.3485, 215.646)
  line L484 (4.6485, 228.346) -> (4.6485, 215.646)
  line L485 (-17.3485, 215.646) -> (-17.3485, 228.346)
  line L486 (-17.3485, 228.346) -> (-6.35, 234.696)
  line L487 (-6.35, 234.696) -> (4.6485, 228.346)
  line L488 (-30.0485, 206.756) -> (-19.05, 213.106)
  line L489 (-8.0515, 206.756) -> (-8.0515, 194.056)
  line L490 (-30.0485, 194.056) -> (-30.0485, 206.756)
  line L491 (-8.0515, 194.056) -> (-19.05, 187.706)
  line L492 (-19.05, 187.706) -> (-30.0485, 194.056)
  line L493 (-19.05, 213.106) -> (-8.0515, 206.756)
  line L494 (4.6485, 258.826) -> (-6.35, 252.476)
  line L495 (-6.35, 252.476) -> (-17.3485, 258.826)
  line L496 (4.6485, 271.526) -> (4.6485, 258.826)
  line L497 (-17.3485, 258.826) -> (-17.3485, 271.526)
  line L498 (-17.3485, 271.526) -> (-6.35, 277.876)
  line L499 (-6.35, 277.876) -> (4.6485, 271.526)
  line L500 (-30.0485, 249.936) -> (-19.05, 256.286)
  line L501 (-8.0515, 249.936) -> (-8.0515, 237.236)
  line L502 (-30.0485, 237.236) -> (-30.0485, 249.936)
  line L503 (-8.0515, 237.236) -> (-19.05, 230.886)
  line L504 (-19.05, 230.886) -> (-30.0485, 237.236)
  line L505 (-19.05, 256.286) -> (-8.0515, 249.936)
  point P0 (0, 0)
  point P1 (-171.45, 27.686)
  point P2 (-158.75, 49.276)
  point P3 (-158.75, 92.456)
  point P4 (-171.45, 70.866)
  point P5 (-158.75, 135.636)
  point P6 (-171.45, 114.046)
  point P7 (-158.75, 178.816)
  point P8 (-171.45, 157.226)
  point P9 (-158.75, 221.996)
  point P10 (-171.45, 200.406)
  point P11 (-133.35, 49.276)
  point P12 (-146.05, 27.686)
  point P13 (-133.35, 92.456)
  point P14 (-146.05, 70.866)
  point P15 (-133.35, 135.636)
  point P16 (-146.05, 114.046)
  point P17 (-133.35, 178.816)
  point P18 (-146.05, 157.226)
  point P19 (-133.35, 221.996)
  point P20 (-146.05, 200.406)
  point P21 (-107.95, 49.276)
  point P22 (-120.65, 27.686)
  point P23 (-107.95, 92.456)
  point P24 (-120.65, 70.866)
  point P25 (-107.95, 135.636)
  point P26 (-120.65, 114.046)
  point P27 (-107.95, 178.816)
  point P28 (-120.65, 157.226)
  point P29 (-107.95, 221.996)
  point P30 (-120.65, 200.406)
  point P31 (-82.55, 49.276)
  point P32 (-95.25, 27.686)
  point P33 (-82.55, 92.456)
  point P34 (-95.25, 70.866)
  point P35 (-82.55, 135.636)
  point P36 (-95.25, 114.046)
  point P37 (-82.55, 178.816)
  point P38 (-95.25, 157.226)
  point P39 (-82.55, 221.996)
  point P40 (-95.25, 200.406)
  point P41 (-57.15, 49.276)
  point P42 (-69.85, 27.686)
  point P43 (-57.15, 92.456)
  point P44 (-69.85, 70.866)
  point P45 (-57.15, 135.636)
  point P46 (-69.85, 114.046)
  point P47 (-57.15, 178.816)
  point P48 (-69.85, 157.226)
  point P49 (-57.15, 221.996)
  point P50 (-69.85, 200.406)
  point P51 (-31.75, 49.276)
  point P52 (-44.45, 27.686)
  point P53 (-31.75, 92.456)
  point P54 (-44.45, 70.866)
  point P55 (-31.75, 135.636)
  point P56 (-44.45, 114.046)
  point P57 (-31.75, 178.816)
  point P58 (-44.45, 157.226)
  point P59 (-31.75, 221.996)
  point P60 (-44.45, 200.406)
  point P61 (-158.75, 265.176)
  point P62 (-171.45, 243.586)
  point P63 (-133.35, 265.176)
  point P64 (-146.05, 243.586)
  point P65 (-107.95, 265.176)
  point P66 (-120.65, 243.586)
  point P67 (-82.55, 265.176)
  point P68 (-95.25, 243.586)
  point P69 (-57.15, 265.176)
  point P70 (-69.85, 243.586)
  point P71 (-31.75, 265.176)
  point P72 (-44.45, 243.586)
  point P73 (-6.35, 49.276)
  point P74 (-19.05, 27.686)
  point P75 (-6.35, 92.456)
  point P76 (-19.05, 70.866)
  point P77 (-6.35, 135.636)
  point P78 (-19.05, 114.046)
  point P79 (-6.35, 178.816)
  point P80 (-19.05, 157.226)
  point P81 (-6.35, 221.996)
  point P82 (-19.05, 200.406)
  point P83 (-6.35, 265.176)
  point P84 (-19.05, 243.586)
  dimension "d286" = 12.7
  dimension "d294" = 12.7
  dimension "d296" = 14.986
  dimension "d297" = 19.05
  dimension "d316" = 2.54
  dimension "d317" = 12.7
  dimension "d320" = 43.18
  dimension "d323" = 25.4
  constraints: 1008 end point, 2 parallel, 1 horizontal, 1 vertical, 1092 other
  measures "d286" distance of L2.end L3.end
  measures "d294" distance of L9.end L10.end
  measures "d296" distance from line of L13 L1.end
  measures "d297" distance from line of L6 L1.end
  measures "d316" vertical distance of L8.end L0.start
  measures "d317" horizontal distance of L8.end L4.end
  measures "d320" distance of L7.end L14.start
  measures "d323" distance of L7.end L62.start
extrude "Extrusion12" cut sketch "Sketch13" against normal blind 11.43 contours A1 L4 L3 L2 L1 L0 | L0 L1 L2 L3 L4 A1 | L7 L8 L9 L10 L11 L12 | L14 L15 L17 L18 L19 L16 | L20 L25 L21 L23 L24 L22 | L26 L27 L29 L30 L31 L28 | L32 L37 L33 L35 L36 L34 | L38 L39 L41 L42 L43 L40 | L44 L49 L45 L47 L48 L46 | L50 L51 L53 L54 L55 L52 | L56 L61 L57 L59 L60 L58 | L62 L63 L65 L66 L67 L64 | L68 L73 L69 L71 L72 L70 | L74 L75 L77 L78 L79 L76 | L80 L85 L81 L83 L84 L82 | L86 L87 L89 L90 L91 L88 | L92 L97 L93 L95 L96 L94 | L98 L99 L101 L102 L103 L100 | L104 L109 L105 L107 L108 L106 | L110 L111 L113 L114 L115 L112 | L116 L121 L117 L119 L120 L118 | L122 L123 L125 L126 L127 L124 | L128 L133 L129 L131 L132 L130 | L134 L135 L137 L138 L139 L136 | L140 L145 L141 L143 L144 L142 | L146 L147 L149 L150 L151 L148 | L152 L157 L153 L155 L156 L154 | L158 L159 L161 L162 L163 L160 | L164 L169 L165 L167 L168 L166 | L170 L171 L173 L174 L175 L172 | L176 L181 L177 L179 L180 L178 | L182 L183 L185 L186 L187 L184 | L188 L193 L189 L191 L192 L190 | L194 L195 L197 L198 L199 L196 | L200 L205 L201 L203 L204 L202 | L206 L207 L209 L210 L211 L208 | L212 L217 L213 L215 L216 L214 | L218 L219 L221 L222 L223 L220 | L224 L229 L225 L227 L228 L226 | L230 L231 L233 L234 L235 L232 | L236 L241 L237 L239 L240 L238 | L242 L243 L245 L246 L247 L244 | L248 L253 L249 L251 L252 L250 | L254 L255 L257 L258 L259 L256 | L260 L265 L261 L263 L264 L262 | L266 L267 L269 L270 L271 L268 | L272 L277 L273 L275 L276 L274 | L278 L279 L281 L282 L283 L280 | L284 L289 L285 L287 L288 L286 | L290 L291 L293 L294 L295 L292 | L296 L301 L297 L299 L300 L298 | L302 L303 L305 L306 L307 L304 | L308 L313 L309 L311 L312 L310 | L314 L315 L317 L318 L319 L316 | L320 L325 L321 L323 L324 L322 | L326 L327 L329 L330 L331 L328 | L332 L337 L333 L335 L336 L334 | L338 L339 L341 L342 L343 L340 | L344 L349 L345 L347 L348 L346 | L350 L351 L353 L354 L355 L352 | L356 L361 L357 L359 L360 L358 | L374 L375 L377 L378 L379 L376 | L380 L385 L381 L383 L384 L382 | L386 L387 L389 L390 L391 L388 | L392 L397 L393 L395 L396 L394 | L398 L399 L401 L402 L403 L400 | L404 L409 L405 L407 L408 L406 | L410 L411 L413 L414 L415 L412 | L416 L421 L417 L419 L420 L418 | L428 L433 L429 L431 L432 L430 | L452 L457 L453 L455 L456 L454 | L464 L469 L465 L467 L468 L466 | L476 L481 L477 L479 L480 L478 | L488 L493 L489 L491 L492 L490
body "Solid1"
